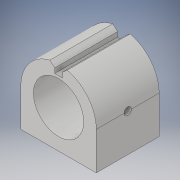
# Autodesk Inventor part: pipe_ruler
Saved by Autodesk Inventor 2019 (Build 230136000, 136)
## iProperties
Created: 2024-08-06
Part Number: pipe_ruler
Material: Generisch
Document SubType Name: Modeling
Designer: nic
Density: 1 g/cm^3
Appearance: Vorgabe
Author: nic
Autodesk Inventor part; units mm, degrees
ref_plane "YZ Plane" through (0, 0, 0) normal (1, 0, 0) x (0, 1, 0)
ref_plane "XZ Plane" through (0, 0, 0) normal (0, 1, 0) x (-1, 0, 0)
ref_plane "XY Plane" through (0, 0, 0) normal (0, 0, 1) x (1, 0, 0)
sketch "Skizze3" plane through (0, 0, 0) normal (0, 0, 1) x (1, 0, 0)
  circle A0 centre (0, 0) radius 10
  arc A1 (15, 0) -> (-15, 0) centre (0, 0) ccw
  line L0 (15, 0) -> (15, -15)
  line L1 (15, -15) -> (-15, -15)
  line L2 (-15, -15) -> (-15, 0)
  line L3 (-15, 15) -> (15, -15) construction
  line L4 (15, 15) -> (-15, -15) construction
  constraints: 10 end point, 2 centre point, 2 midpoint, 2 point on circle, 1 coincident, 1 parallel
extrude "Extrusion2" add sketch "Skizze3" along normal blind 25
sketch "Skizze4" plane through (0, 0, 25) normal (0, 0, 1) x (1, 0, 0)
  circle A0 centre (0, 0) radius 10 construction
  line L0 (15, -15) -> (15, 0) construction
  arc A1 (15, 0) -> (-15, 0) centre (0, 0) ccw construction
  line L1 (-15, 0) -> (-15, -15) construction
  line L2 (-15, -15) -> (15, -15) construction
  line L3 (-1.5, 19) -> (1.5, 19)
  line L4 (1.5, 19) -> (1.5, 11)
  line L5 (1.5, 11) -> (-1.5, 11)
  line L6 (-1.5, 11) -> (-1.5, 19)
  arc A2 (15, 0) -> (-15, 0) centre (0, 0) ccw projected
  line L7 (-1.5, 19) -> (1.5, 11) construction
  line L8 (1.5, 19) -> (-1.5, 11) construction
  point P0 (0, 15)
  dimension "d9" = 3
  dimension "d10" = 8
  constraints: 12 end point, 2 midpoint, 2 parallel, 2 point on circle, 1 horizontal, 1 perpendicular
  measures "d9" distance of L4.end L5.end
  measures "d10" distance of L3.end L4.end
extrude "Extrusion3" cut sketch "Skizze4" against normal through all
chamfer "Fase1" distance 2 angle 45 2 edges at (-1.5, 14.9248, 12.5) (1.5, 14.9248, 12.5)
sketch "Skizze5" plane through (15, -15, 0) normal (1, 0, 0) x (0, 0, -1)
  line L0 (0, 15) -> (-25, 15) projected
  circle A0 centre (-12.5, 15) radius 1.45
  dimension "d16" = 2.9
  constraints: 1 centre point, 1 midpoint
  measures "d16" diameter of A0
extrude "Extrusion4" cut sketch "Skizze5" against normal blind 6
